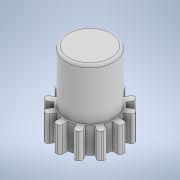
# Autodesk Inventor part: Gear1
Saved by Autodesk Inventor 2022 (Build 260153000, 153)
## iProperties
Created: 2021-09-18
Part Number: Gear1
Material: Generic
Document SubType Name: Modeling
Designer: marcu
Density: 1 g/cm^3
Appearance: Default
Author: marcu
Autodesk Inventor part; units mm, degrees
ref_plane "YZ Plane" through (0, 0, 0) normal (1, 0, 0) x (0, 1, 0)
ref_plane "XZ Plane" through (0, 0, 0) normal (0, 1, 0) x (-1, 0, 0)
ref_plane "XY Plane" through (0, 0, 0) normal (0, 0, 1) x (1, 0, 0)
sketch "Sketch1" plane through (0, 0, 0) normal (0, 1, 0) x (-1, 0, 0)
  circle A0 centre (0, 0) radius 2.921
  dimension "d0" = 5.842
  constraints: 1 centre point, 1 coincident
  measures "d0" diameter of A0
extrude "Extrusion1" add sketch "Sketch1" along normal blind 6.35
sketch "Sketch2" plane through (0, 0, 0) normal (0, -1, 0) x (1, 0, 0)
  circle A0 centre (0, 0) radius 2.921
  line L0 (-4.1275, -0.4128) -> (4.1275, -0.4128)
  line L1 (4.1275, -0.4128) -> (4.1275, 0.4128)
  line L2 (4.1275, 0.4128) -> (-4.1275, 0.4128)
  line L3 (-4.1275, 0.4128) -> (-4.1275, -0.4128)
  line L4 (-4.1275, -0.4128) -> (4.1275, 0.4128) construction
  line L5 (4.1275, -0.4128) -> (-4.1275, 0.4128) construction
  line L6 (3.7809, 1.7063) -> (3.3681, 2.4212)
  line L7 (-3.3681, -2.4212) -> (3.7809, 1.7063)
  line L8 (3.3681, 2.4212) -> (-3.7809, -1.7063)
  line L9 (-3.7809, -1.7063) -> (-3.3681, -2.4212)
  line L10 (2.4212, 3.3681) -> (1.7063, 3.7809)
  line L11 (-1.7063, -3.7809) -> (2.4212, 3.3681)
  line L12 (1.7063, 3.7809) -> (-2.4212, -3.3681)
  line L13 (-2.4212, -3.3681) -> (-1.7063, -3.7809)
  line L14 (0.4128, 4.1275) -> (-0.4127, 4.1275)
  line L15 (0.4127, -4.1275) -> (0.4128, 4.1275)
  line L16 (-0.4127, 4.1275) -> (-0.4128, -4.1275)
  line L17 (-0.4128, -4.1275) -> (0.4127, -4.1275)
  line L18 (-1.7063, 3.7809) -> (-2.4212, 3.3681)
  line L19 (2.4212, -3.3681) -> (-1.7063, 3.7809)
  line L20 (-2.4212, 3.3681) -> (1.7063, -3.7809)
  line L21 (1.7063, -3.7809) -> (2.4212, -3.3681)
  line L22 (-3.3681, 2.4212) -> (-3.7809, 1.7063)
  line L23 (3.7809, -1.7063) -> (-3.3681, 2.4212)
  line L24 (-3.7809, 1.7063) -> (3.3681, -2.4212)
  line L25 (3.3681, -2.4212) -> (3.7809, -1.7063)
  line L26 (-4.1275, 0.4128) -> (-4.1275, -0.4127)
  line L27 (4.1275, 0.4127) -> (-4.1275, 0.4128)
  line L28 (-4.1275, -0.4127) -> (4.1275, -0.4128)
  line L29 (4.1275, -0.4128) -> (4.1275, 0.4127)
  line L30 (-3.7809, -1.7063) -> (-3.3681, -2.4212)
  line L31 (3.3681, 2.4212) -> (-3.7809, -1.7063)
  line L32 (-3.3681, -2.4212) -> (3.7809, 1.7063)
  line L33 (3.7809, 1.7063) -> (3.3681, 2.4212)
  line L34 (-2.4212, -3.3681) -> (-1.7063, -3.7809)
  line L35 (1.7063, 3.7809) -> (-2.4212, -3.3681)
  line L36 (-1.7063, -3.7809) -> (2.4212, 3.3681)
  line L37 (2.4212, 3.3681) -> (1.7063, 3.7809)
  line L38 (-0.4128, -4.1275) -> (0.4127, -4.1275)
  line L39 (-0.4127, 4.1275) -> (-0.4128, -4.1275)
  line L40 (0.4127, -4.1275) -> (0.4128, 4.1275)
  line L41 (0.4128, 4.1275) -> (-0.4127, 4.1275)
  line L42 (1.7063, -3.7809) -> (2.4212, -3.3681)
  line L43 (-2.4212, 3.3681) -> (1.7063, -3.7809)
  line L44 (2.4212, -3.3681) -> (-1.7063, 3.7809)
  line L45 (-1.7063, 3.7809) -> (-2.4212, 3.3681)
  line L46 (3.3681, -2.4212) -> (3.7809, -1.7063)
  line L47 (-3.7809, 1.7063) -> (3.3681, -2.4212)
  line L48 (3.7809, -1.7063) -> (-3.3681, 2.4212)
  line L49 (-3.3681, 2.4212) -> (-3.7809, 1.7063)
  circle A1 centre (0, 0) radius 3.175
  circle A2 centre (0, 0) radius 3.175
  point P0 (2.9327, -1.2166)
  point P1 (3.1481, -0.4127)
  point P2 (3.1481, 0.4128)
  point P3 (2.9327, 1.2166)
  point P4 (2.5199, 1.9315)
  point P5 (1.9315, 2.5199)
  point P6 (1.2166, 2.9327)
  point P7 (0.4128, 3.1481)
  point P8 (-0.4128, 3.1481)
  point P9 (-1.2166, 2.9327)
  point P10 (-1.9315, 2.5199)
  point P11 (-2.5199, 1.9315)
  point P12 (-2.9327, 1.2166)
  point P13 (-3.1481, 0.4127)
  point P14 (-3.1481, -0.4128)
  point P15 (-2.9327, -1.2166)
  point P16 (-2.5199, -1.9315)
  point P17 (-1.9315, -2.5199)
  point P18 (-1.2166, -2.9327)
  point P19 (-0.4128, -3.1481)
  point P20 (0.4127, -3.1481)
  point P21 (1.2166, -2.9327)
  point P22 (1.9315, -2.5199)
  point P23 (2.5199, -1.9315)
  dimension "d5" = 8.255
  dimension "d6" = 0.8255
  dimension "d7" = 360
  constraints: 100 end point, 2 centre point, 2 midpoint, 2 parallel, 1 coincident, 1 horizontal, 1 perpendicular, 100 other
  measures "d5" distance of L2.end L1.end
  measures "d6" distance of L1.end L0.end
extrude "Extrusion2" add sketch "Sketch2" along normal blind 3.175
fillet "Fillet1" radius 0.3175 2 edges at (2.4212, -1.5875, 3.3681) (1.7063, -1.5875, 3.7809)
pattern_circular "Circular Pattern1" count 12 over 360 about axis through (0, 0, 0) along (0, 1, 0) of "Fillet1", "Extrusion1"
fillet "Fillet2" radius 0.3175 1 edges at (2.921, 6.35, 0)
sketch "Sketch3" plane through (0, -3.175, 0) normal (0, -1, 0) x (1, 0, 0)
  line L0 (-1.5875, -1.5875) -> (1.5875, -1.5875)
  line L1 (1.5875, -1.5875) -> (1.5875, 1.5875)
  line L2 (1.5875, 1.5875) -> (-1.5875, 1.5875)
  line L3 (-1.5875, 1.5875) -> (-1.5875, -1.5875)
  line L4 (-1.5875, -1.5875) -> (1.5875, 1.5875) construction
  line L5 (1.5875, -1.5875) -> (-1.5875, 1.5875) construction
  point P0 (0, 0)
  dimension "d15" = 3.175
  dimension "d16" = 3.175
  constraints: 12 end point, 2 midpoint, 2 parallel, 1 horizontal, 1 perpendicular
  measures "d15" distance of L2.end L1.end
  measures "d16" distance of L1.end L0.end
extrude "Extrusion3" cut sketch "Sketch3" against normal blind 3.175
body "Solid1"
